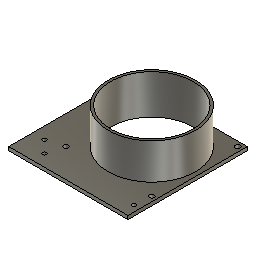
fan mount down v2 (Autodesk Fusion 360 design; units mm, degrees)
Autodesk Fusion 360 part; units mm, degrees
sketch "Skizze1" plane through (0, 0, 0) normal (0, 0, 1) x (1, 0, 0)
  line L0 (0, 0) -> (100, 0)
  line L1 (100, 0) -> (100, 100)
  line L2 (100, 100) -> (0, 100)
  line L3 (0, 100) -> (0, 0)
  line L4 (100, 100) -> (20, 100)
  line L5 (20, 100) -> (20, 20)
  line L6 (20, 20) -> (100, 20)
  line L7 (100, 20) -> (100, 100)
  circle A0 centre (96, 24) radius 2
  circle A1 centre (24, 96) radius 2
  circle A2 centre (96, 96) radius 2
  circle A3 centre (24, 24) radius 2
  circle A4 centre (60, 60) radius 34.5
  dimension "d1" = 100
  dimension "d2" = 100
  dimension "d3" = 80
  dimension "d4" = 80
  dimension "d5" = 72
  dimension "d6" = 72
  dimension "d9" = 4
  dimension "d10" = 4
  dimension "d11" = 4
  dimension "d12" = 4
  dimension "d13" = 69
  constraint horizontal L0
  constraint vertical L1
  constraint horizontal L2
  constraint vertical L3
  constraint coincident L0.start L3.end
  constraint horizontal L4
  constraint vertical L5
  constraint horizontal L6
  constraint vertical L7
  measures "d1" distance of L0.start L0.end
  measures "d2" distance of L0.start L2.end
  measures "d3" distance of L1.end L4.end
  measures "d4" distance of L1.end L6.end
  measures "d5" distance of A1.centre A2.centre
  measures "d6" distance of A1.centre A3.centre
  measures "d9" diameter of A0
  measures "d10" diameter of A1
  measures "d11" diameter of A2
  measures "d12" diameter of A3
  measures "d13" diameter of A4
extrude "Extrusion1" add sketch "Skizze1" along normal blind 3
sketch "Skizze2" plane through (0, 0, 3) normal (0, 0, 1) x (-1, 0, 0)
  circle A0 centre (-24, -24) radius 2
  circle A1 centre (-60, -60) radius 34.5
  circle A2 centre (-96, -24) radius 2
  circle A3 centre (-96, -96) radius 2
  circle A4 centre (-24, -96) radius 2
  line L0 (-100, 0) -> (-100, -100)
  line L1 (-100, -100) -> (0, -100)
  line L2 (0, -100) -> (0, 0)
  line L3 (0, 0) -> (-100, 0)
  circle A5 centre (-95, -10) radius 1.6
  circle A6 centre (-20, -10) radius 1.6
  circle A7 centre (-10, -20) radius 1.6
  circle A8 centre (-10, -95) radius 1.6
  dimension "d17" = 3.2
  dimension "d18" = 3.2
  dimension "d19" = 3.2
  dimension "d20" = 3.2
  measures "d17" diameter of A5
  measures "d18" diameter of A6
  measures "d19" diameter of A7
  measures "d20" diameter of A8
extrude "Extrusion2" cut sketch "Skizze2" against normal blind 10 contours A5 | A6 | A7 | A8
sketch "Skizze3" plane through (0, 0, 3) normal (0, 0, 1) x (-1, 0, 0)
  circle A0 centre (-10, -20) radius 1.6
  circle A1 centre (-95, -10) radius 1.6
  circle A2 centre (-20, -10) radius 1.6
  circle A3 centre (-10, -95) radius 1.6
  circle A4 centre (-96, -96) radius 2
  circle A5 centre (-24, -24) radius 2
  circle A6 centre (-24, -96) radius 2
  circle A7 centre (-60, -60) radius 34.5
  circle A8 centre (-96, -24) radius 2
  line L0 (-100, 0) -> (-100, -100)
  line L1 (-100, -100) -> (0, -100)
  line L2 (0, -100) -> (0, 0)
  line L3 (0, 0) -> (-100, 0)
  circle A9 centre (-60, -60) radius 36.5
  dimension "d23" = 73
  constraint concentric A7 A9
  measures "d23" diameter of A9
extrude "Extrusion3" add sketch "Skizze3" along normal blind 30 contours A9
